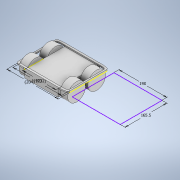
# Autodesk Inventor part: Деталь18
Saved by Autodesk Inventor 2020 (Build 240168000, 168)
## iProperties
Created: 2022-07-17
Part Number: Деталь18
Material: Типовые
Document SubType Name: Modeling
Designer: akapu
Density: 1 g/cm^3
Appearance: По умолчанию
Author: akapu
Autodesk Inventor part; units mm, degrees
ref_plane "YZ Plane" through (0, 0, 0) normal (1, 0, 0) x (0, 1, 0)
ref_plane "XZ Plane" through (0, 0, 0) normal (0, 1, 0) x (-1, 0, 0)
ref_plane "XY Plane" through (0, 0, 0) normal (0, 0, 1) x (1, 0, 0)
sketch "Эскиз1" plane through (0, 0, 0) normal (0, 1, 0) x (-1, 0, 0)
  line L0 (0, 0) -> (-132, 0)
  line L1 (-132, 0) -> (-132, -165.5)
  line L2 (-132, -165.5) -> (0, -165.5)
  line L3 (0, -165.5) -> (0, 0)
  line L4 (0, 0) -> (-132, 0)
  line L5 (-132, 0) -> (-132, -8)
  line L6 (-132, -8) -> (0, -8)
  line L7 (0, -8) -> (0, 0)
  line L8 (0, -165.5) -> (-132, -165.5)
  line L9 (-132, -165.5) -> (-132, -157.5)
  line L10 (-132, -157.5) -> (0, -157.5)
  line L11 (0, -157.5) -> (0, -165.5)
  line L12 (0, 0) -> (0, -43)
  line L13 (0, -43) -> (0, -8)
  line L14 (0, -8) -> (30, -8)
  line L15 (30, -8) -> (30, -78)
  line L16 (30, -78) -> (0, -78)
  line L17 (0, -78) -> (0, -8)
  line L18 (0, -157.5) -> (30, -157.5)
  line L19 (30, -157.5) -> (30, -87.5)
  line L20 (30, -87.5) -> (0, -87.5)
  line L21 (0, -87.5) -> (0, -157.5)
  line L22 (-132, -8) -> (-162, -8)
  line L23 (-162, -8) -> (-162, -78)
  line L24 (-162, -78) -> (-132, -78)
  line L25 (-132, -78) -> (-132, -8)
  line L26 (-132, -157.5) -> (-162, -157.5)
  line L27 (-162, -157.5) -> (-162, -87.5)
  line L28 (-162, -87.5) -> (-132, -87.5)
  line L29 (-132, -87.5) -> (-132, -157.5)
  dimension "d0" = 132
  dimension "d1" = 165.5
  dimension "d2" = 8
  dimension "d3" = 8
  dimension "d4" = 43
  dimension "d5" = 35
  dimension "d6" = 30
  dimension "d7" = 70
  dimension "d8" = 30
  dimension "d9" = 70
  dimension "d10" = 30
  dimension "d11" = 70
  dimension "d12" = 30
  dimension "d13" = 70
  constraints: 60 end point, 14 parallel, 7 horizontal, 7 perpendicular, 3 point on line, 1 collinear
  measures "d0" distance of L2.end L1.end
  measures "d1" distance of L1.end L0.end
  measures "d2" distance of L5.end L4.end
  measures "d3" distance of L8.end L9.end
  measures "d4" distance of L0.start L12.end
  measures "d5" distance of L12.end L6.end
  measures "d6" distance of L15.end L16.end
  measures "d7" distance of L14.end L15.end
  measures "d8" distance of L20.end L19.end
  measures "d9" distance of L19.end L18.end
  measures "d10" distance of L24.end L23.end
  measures "d11" distance of L23.end L22.end
  measures "d12" distance of L27.end L28.end
  measures "d13" distance of L26.end L27.end
extrude "Выдавливание1" add sketch "Эскиз1" along normal blind 30 contours L3 L6 L1 L0 | L3 L10 L1 L6 | L10 L3 L2 L1
sketch "Эскиз2" plane through (132, 0, 0) normal (1, 0, 0) x (0, 0, -1)
  line L0 (0, 0) -> (0, 30) projected
  line L1 (165.5, 0) -> (165.5, 30) projected
  line L2 (165.5, 0) -> (0, 0) projected
  line L3 (0, 0) -> (43, 0)
  line L4 (43, 0) -> (43, 4.5763)
  line L5 (43, 4.5763) -> (43, 30)
  line L6 (43, 0) -> (43, 12.5)
  line L7 (165.5, 0) -> (122.5, 0)
  line L8 (122.5, 0) -> (122.5, 12.5)
  line L9 (122.5, 12.5) -> (43, 12.5)
  circle A0 centre (43, 12.5) radius 35
  circle A1 centre (122.5, 12.5) radius 35
  dimension "d24" = 43
  dimension "d25" = 12.5
  dimension "d26" = 43
  dimension "d27" = 70
  dimension "d28" = 70
  constraints: 14 end point, 4 point on line, 2 centre point, 2 coincident, 2 perpendicular
  measures "d24" distance of L0.start L3.end
  measures "d25" distance of L3.end L6.end
  measures "d26" distance of L1.start L7.end
  measures "d27" diameter of A0
  measures "d28" diameter of A1
extrude "Выдавливание2" add sketch "Эскиз2" along normal blind 30 contours A1 L2 | L2 L8 L9 A1 | L2 A1 L9 L8 | A0 L2 | L2 L4 L5 L9 A0 | L2 A0 L9 L5 L4
sketch "Эскиз3" plane through (0, 0, -165.5) normal (-1, 0, 0) x (0, 0, 1)
  circle A0 centre (122.5, 12.5) radius 35 projected
  circle A1 centre (122.5, 12.5) radius 35
  arc A2 (10.3083, 0) -> (75.6917, 0) centre (43, 12.5) ccw projected
  circle A3 centre (43, 12.5) radius 35
  point P0 (165.5, 0)
  point P1 (122.5, 15)
  point P2 (43, 15)
  point P3 (75.6917, 0)
  constraints: 2 centre point, 2 coincident
extrude "Выдавливание3" add sketch "Эскиз3" along normal blind 30
sketch "Эскиз4" plane through (0, 30, 0) normal (0, 1, 0) x (1, 0, 0)
  line L0 (-30, 78) -> (-30, 8) projected
  line L1 (-36, 8) -> (-36, 0)
  line L2 (132, 165.5) -> (0, 165.5) projected
  line L3 (-36, 0) -> (0, 0)
  line L4 (0, 0) -> (0, 165.5)
  line L5 (0, 165.5) -> (-36, 165.5)
  line L6 (-36, 165.5) -> (-36, 0)
  line L7 (132, 152.8109) -> (132, 165.5) projected
  line L8 (132, 165.5) -> (168, 165.5)
  line L9 (168, 165.5) -> (168, 0)
  line L10 (168, 0) -> (132, 0)
  line L11 (132, 0) -> (132, 165.5)
  line L12 (0, 8) -> (-30, 8) projected
  line L13 (-30, 157.5) -> (-30, 87.5) projected
  line L14 (0, 8) -> (-30, 8)
  line L15 (-30, 8) -> (-30, 157.5)
  line L16 (-30, 157.5) -> (0, 157.5)
  line L17 (0, 157.5) -> (0, 8)
  line L18 (162, 8) -> (162, 78) projected
  line L19 (132, 157.5) -> (162, 157.5)
  line L20 (162, 157.5) -> (162, 8)
  line L21 (162, 8) -> (132, 8)
  line L22 (132, 8) -> (132, 157.5)
  line L23 (168, 0) -> (-36, 0)
  line L24 (-36, 0) -> (-36, 165.5)
  line L25 (-36, 165.5) -> (168, 165.5)
  line L26 (168, 165.5) -> (168, 0)
  line L27 (0, 157.5) -> (132, 157.5)
  line L28 (132, 157.5) -> (132, 165.5)
  line L29 (132, 165.5) -> (0, 165.5)
  line L30 (0, 165.5) -> (0, 157.5)
  line L31 (0, 8) -> (0, 12.6891) projected
  line L32 (132, 0) -> (0, 0)
  line L33 (0, 0) -> (0, 8)
  line L34 (0, 8) -> (132, 8)
  line L35 (132, 8) -> (132, 0)
  line L36 (168, 165.5) -> (165, 165.5)
  line L37 (165, 165.5) -> (165, 161.5)
  line L38 (165, 161.5) -> (168, 161.5)
  line L39 (168, 161.5) -> (168, 165.5)
  line L40 (168, 0) -> (165, 0)
  line L41 (165, 0) -> (165, 4)
  line L42 (165, 4) -> (168, 4)
  line L43 (168, 4) -> (168, 0)
  line L44 (-36, 0) -> (-33, 0)
  line L45 (-33, 0) -> (-33, 4)
  line L46 (-33, 4) -> (-36, 4)
  line L47 (-36, 4) -> (-36, 0)
  line L48 (-36, 165.5) -> (-33, 165.5)
  line L49 (-33, 165.5) -> (-33, 161.5)
  line L50 (-33, 161.5) -> (-36, 161.5)
  line L51 (-36, 161.5) -> (-36, 165.5)
  line L52 (0, 165.5) -> (0, 155.1917) projected
  spline S0 degree 2 poles (0, 165.5) (-35.5316, 165.8812) (-36, 157.5) knots 0 0 0 1 1 1
  spline S1 degree 2 poles (132, 165.5) (167.5316, 165.8812) (168, 157.5) knots 0 0 0 1 1 1
  spline S2 degree 2 poles (132, 0) (167.5316, -0.3812) (168, 8) knots 0 0 0 1 1 1
  line L53 (0, 0) -> (132, 0) projected
  spline S3 degree 2 poles (0, 0) (-35.5316, -0.3812) (-36, 8) knots 0 0 0 1 1 1
  line L54 (-30, 8) -> (-27, 8)
  line L55 (-27, 8) -> (-27, 10)
  line L56 (-27, 10) -> (-30, 10)
  line L57 (-30, 10) -> (-30, 8)
  spline S4 degree 2 poles (0, 8) (-28.3192, 6.9002) (-30, 12.6891) knots 0 0 0 1 1 1
  line L58 (162, 8) -> (159, 8)
  line L59 (159, 8) -> (159, 10)
  line L60 (159, 10) -> (162, 10)
  line L61 (162, 10) -> (162, 8)
  line L62 (162, 157.5) -> (159, 157.5)
  line L63 (159, 157.5) -> (159, 155.5)
  line L64 (159, 155.5) -> (162, 155.5)
  line L65 (162, 155.5) -> (162, 157.5)
  line L66 (-30, 157.5) -> (-27, 157.5)
  line L67 (-27, 157.5) -> (-27, 155.5)
  line L68 (-27, 155.5) -> (-30, 155.5)
  line L69 (-30, 155.5) -> (-30, 157.5)
  spline S5 degree 2 poles (-30, 152.8109) (-28.3192, 158.5998) (0, 157.5) knots 0 0 0 1 1 1
  line L70 (162, 87.5) -> (162, 157.5) projected
  spline S6 degree 2 poles (132, 157.5) (160.3192, 158.5998) (162, 152.8109) knots 0 0 0 1 1 1
  spline S7 degree 2 poles (132, 8) (160.3192, 6.9002) (162, 12.6891) knots 0 0 0 1 1 1
  point P0 (0, 10.3083)
  point P1 (162, 152.8109)
  point P2 (137.9176, 0)
  point P3 (168, 8)
  point P4 (168, 157.5)
  point P5 (137.9176, 165.5)
  point P6 (-5.9176, 165.5)
  point P7 (-36, 157.5)
  point P8 (-5.9176, 0)
  point P9 (-30, 12.6891)
  point P10 (-30, 152.8109)
  dimension "d30" = 36
  dimension "d31" = 3
  dimension "d32" = 3
  dimension "d33" = 3
  dimension "d34" = 2
  dimension "d35" = 3
  dimension "d36" = 2
  dimension "d37" = 3
  dimension "d38" = 2
  constraints: 122 end point, 30 parallel, 16 point on line, 15 horizontal, 15 perpendicular, 24 other
  measures "d30" distance of L9.end L10.end
  measures "d31" distance of L38.end L37.end
  measures "d32" distance of L46.end L45.end
  measures "d33" distance of L56.end L55.end
  measures "d34" distance of L55.end L54.end
  measures "d35" distance of L59.end L60.end
  measures "d36" distance of L58.end L59.end
  measures "d37" distance of L64.end L63.end
  measures "d38" distance of L63.end L62.end
extrude "Выдавливание4" add sketch "Эскиз4" along normal blind 5 contours L0 L12 S4 L4 L3 S3 L6 S0 L5 S5 L16 L13 L15 | S4 L56 L0 | L56 L55 L12 L0 | S4 L12 L55 | L13 L68 S5 | L13 L16 L67 L68 | L67 L16 S5 | L34 L11 L23 L4 | S7 L21 L18 L20 L19 S6 L7 L8 S1 L9 S2 L10 L11 | L4 L2 L7 L27 | S7 L59 L21 | L59 L60 L18 L21 | S7 L18 L60 | L19 L63 S6 | L19 L20 L64 L63 | L64 L20 S6
sketch "Эскиз6" plane through (0, 30, 0) normal (0, 1, 0) x (1, 0, 0)
  line L0 (168, 8) -> (168, 157.5) projected
  line L1 (-36, 157.5) -> (-36, 8) projected
  line L2 (162, 16.1905) -> (162, 69.8095) projected
  line L3 (-30, 69.8095) -> (-30, 16.1905) projected
  line L4 (132, 12.6891) -> (132, 73.3109) projected
  line L5 (0, 73.3109) -> (0, 12.6891) projected
  line L6 (187.3576, 0) -> (377.3576, 0)
  line L7 (377.3576, 0) -> (377.3576, 165.5)
  line L8 (377.3576, 165.5) -> (187.3576, 165.5)
  line L9 (187.3576, 165.5) -> (187.3576, 0)
  point P0 (0, 0)
  dimension "d41" = 204
  dimension "d42" = 192
  dimension "d43" = 132
  dimension "d44" = 190
  dimension "d45" = 165.5
  constraints: 8 end point, 2 parallel, 1 horizontal, 1 perpendicular
  measures "d41" distance between parallel lines of L0 L1
  measures "d42" distance between parallel lines of L2 L3
  measures "d43" distance between parallel lines of L4 L5
  measures "d44" distance of L8.end L7.end
  measures "d45" distance of L7.end L6.end
